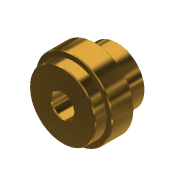
# Autodesk Inventor part: cyl head
Saved by Autodesk Inventor 2022 Beta2 (Build 260130000, 130) ContinuousBuild 0
## iProperties
Shininess: 27.0
Length Units: 11272
Angle Units: 11279
Time Units: 11290
Mass Units: 11286
Length Display Precision: 3
Angle Display Precision: 2
Created: 2001-07-19
Part Number: cyl head
Document SubType Name: Modeling
Designer: smithga
Density: 1 g/cm^3
Material: Generic
Appearance: Brass - Satin
Density: 0.0
Volumn: 0.0
Area: 0.0
PropertySet Name: Model Information
Control State: 0
Master: False
Checked Out: False
Author: smithga
Autodesk Inventor part; units mm, degrees
ref_plane "YZ Plane" through (0, 0, 0) normal (1, 0, 0) x (0, 1, 0)
ref_plane "XZ Plane" through (0, 0, 0) normal (0, 1, 0) x (-1, 0, 0)
ref_plane "XY Plane" through (0, 0, 0) normal (0, 0, 1) x (1, 0, 0)
sketch "Sketch1" plane through (0, 0, 0) normal (0, 0, 1) x (1, 0, 0)
  circle A0 centre (0, 0) radius 7.9375
  circle A1 centre (0, 0) radius 3.175
  constraints: 2 centre point, 1 coincident
extrude "Extrusion1" add sketch "Sketch1" along normal blind 6.35
sketch "Sketch2" plane through (0, 0, 6.35) normal (0, 0, 1) x (1, 0, 0)
  circle A0 centre (0, 0) radius 3.175 projected
  circle A1 centre (0, 0) radius 7.9375 projected
  circle A2 centre (0, 0) radius 11.1125
  constraints: 2 coincident, 1 centre point
extrude "Extrusion2" add sketch "Sketch2" along normal blind 6.35 contours A1 | A2
sketch "Sketch3" plane through (0, 0, 12.7) normal (0, 0, 1) x (1, 0, 0)
  circle A0 centre (0, 0) radius 3.175 projected
  circle A1 centre (0, 0) radius 11.1125 projected
  circle A2 centre (0, 0) radius 9.525
  constraints: 1 centre point, 1 coincident
extrude "Extrusion3" add sketch "Sketch3" along normal blind 3.175 contours A2
chamfer "Chamfer1" distance 0.254 angle 45 6 edges at (-9.525, 0, 15.875) (-3.175, 0, 15.875) (-11.1125, 0, 12.7) (-11.1125, 0, 6.35) (-7.9375, 0, 0) (-3.175, 0, 0)
body "Solid1"
